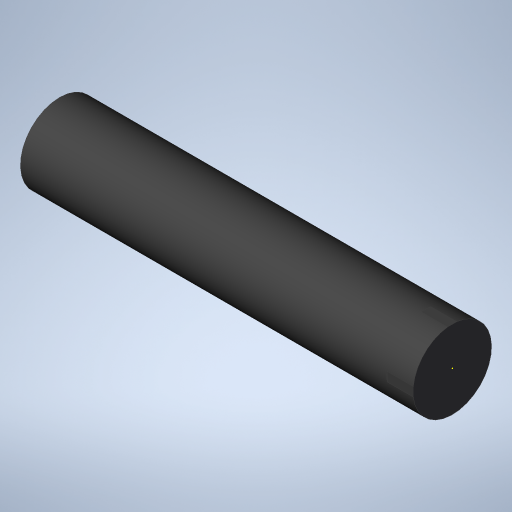
# Autodesk Inventor part: pin
Saved by Autodesk Inventor 2024.3 (Build 283343000, 343)
## iProperties
Created: 2025-06-26
Part Number: pin
Material: Generic
Document SubType Name: Modeling
Designer: ajclo
Density: 1 g/cm^3
Appearance: Default
Mass: 0.105884 g
Surface Area: 1.5546 cm^2
Volume: 0.105884 cm^3
Author: ajclo
Autodesk Inventor part; units mm, degrees
ref_plane "YZ Plane" through (0, 0, 0) normal (1, 0, 0) x (0, 1, 0)
ref_plane "XZ Plane" through (0, 0, 0) normal (0, 1, 0) x (-1, 0, 0)
ref_plane "XY Plane" through (0, 0, 0) normal (0, 0, 1) x (1, 0, 0)
sketch "Sketch1" plane through (0, 0, 0) normal (1, 0, 0) x (0, 1, 0)
  circle A0 centre (-0.038, 0) radius 1.5
  point P0 (0, 0)
  dimension "d0" = 3
  constraints: 1 centre point
  measures "d0" diameter of A0
extrude "Extrusion1" add sketch "Sketch1" along normal blind 15
sketch "Sketch2" plane through (15, -0.038, 0) normal (1, 0, 0) x (0, 0, -1)
  circle A0 centre (0, 0) radius 1.5 projected
  line L0 (-0.1729, 1.49) -> (0.1729, 1.49)
  point P0 (0, 0.038)
  point P1 (0, 1.49)
  dimension "d3" = 1.49
  constraints: 2 end point, 2 point on circle, 1 horizontal, 1 midpoint
  measures "d3" distance of A0.centre point (0, 1.49)
extrude "Extrusion2" cut sketch "Sketch2" against normal blind 1 contours L0 A0 picked at (-0.0192, 1.493)
sketch "Sketch3" plane through (15, 0, 0) normal (1, 0, 0) x (0, 0, -1)
  point P0 (0, 0)
sketch "Sketch4" plane through (15, 0, 0) normal (1, 0, 0) x (0, 0, -1)
  arc A0 (-0.1729, 1.452) -> (0.1729, 1.452) centre (0, -0.038) ccw projected
  line L0 (-1.49, 0.135) -> (-1.49, -0.2109)
  line L1 (0.1729, 1.452) -> (-0.1729, 1.452) projected
  point P0 (0, 0)
  point P1 (-1.49, -0.038)
  dimension "d6" = 1.49
  constraints: 2 end point, 2 point on circle, 1 midpoint, 1 perpendicular
  measures "d6" horizontal distance of point (0, 0) point (-1.49, -0.038)
extrude "Extrusion3" cut sketch "Sketch4" against normal blind 1 contours L0 A0
body "Solid1"
